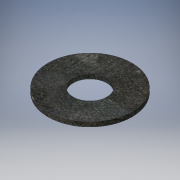
# Autodesk Inventor part: washer2_5x1_0
Saved by Autodesk Inventor 2019.3 (Build 233278000, 278)
## iProperties
Created: 2019-03-05
Part Number: washer2_5x1_0
Material: Steel
Document SubType Name: Modeling
Designer: steele
Density: 7.85 g/cm^3
Appearance: Plate
Mass: 74.2588 g
Surface Area: 63.1358 cm^2
Volume: 9.45972 cm^3
Author: steele
Autodesk Inventor part; units mm, degrees
ref_plane "YZ Plane" through (0, 0, 0) normal (1, 0, 0) x (0, 1, 0)
ref_plane "XZ Plane" through (0, 0, 0) normal (0, 1, 0) x (-1, 0, 0)
ref_plane "XY Plane" through (0, 0, 0) normal (0, 0, 1) x (1, 0, 0)
sketch "Sketch1" plane through (0, 0, 0) normal (0, 1, 0) x (-1, 0, 0)
  circle A0 centre (0, 0) radius 12.7
  circle A1 centre (0, 0) radius 31.75
  dimension "id" = 25.4
  dimension "od" = 63.5
  constraints: 2 centre point, 2 coincident
  measures "id" diameter of A0
  measures "od" diameter of A1
extrude "Extrusion1" add sketch "Sketch1" against normal blind 3.556
body "Solid1"
